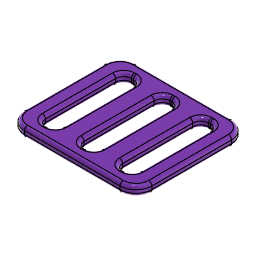
TriGlide v3 (Autodesk Fusion 360 design; units mm, degrees)
Autodesk Fusion 360 part; units mm, degrees
other "Base Mesh Feature1"
sketch "Sketch1" plane through (0, 0, 0) normal (0, 0, 1) x (1, 0, 0)
  line L0 (-12.5, 12.5) -> (-12.5, -12.5)
  line L1 (-7.5, -17.5) -> (22.5, -17.5)
  line L2 (27.5, -12.5) -> (27.5, 12.5)
  line L3 (22.5, 17.5) -> (-7.5, 17.5)
  arc A0 (-7.5, 17.5) -> (-12.5, 12.5) centre (-7.5, 12.5) ccw
  arc A1 (27.5, 12.5) -> (22.5, 17.5) centre (22.5, 12.5) ccw
  arc A2 (-12.5, -12.5) -> (-7.5, -17.5) centre (-7.5, -12.5) ccw
  arc A3 (22.5, -17.5) -> (27.5, -12.5) centre (22.5, -12.5) ccw
  dimension "d1" = 5
  dimension "outerFillet" = 5
  dimension "d3" = 5
  dimension "d4" = 5
  dimension "d17" = 40
  dimension "d18" = 12.5
  constraint vertical L0
  constraint perpendicular L0 L1
  constraint perpendicular L1 L2
  constraint perpendicular L2 L3
  constraint tangent L0 A0
  constraint tangent L3 A0
  constraint tangent L2 A1
  constraint tangent L3 A1
  constraint tangent L0 A2
  constraint tangent L1 A2
  constraint tangent L1 A3
  constraint tangent L2 A3
  measures "d1" radius of A0
  measures "outerFillet" radius of A1
  measures "d3" radius of A2
  measures "d4" radius of A3
  measures "d17" distance of L0 L2
  measures "d18" distance of origin L0
sketch "Sketch2" plane through (0, 0, 0) normal (0, 0, 1) x (1, 0, 0)
  line L0 (-4.9, 13.5) -> (-4.3, 13.5)
  line L1 (-4.9, -13.5) -> (-4.3, -13.5)
  line L2 (-7.4, 11) -> (-7.4, -11)
  line L3 (-1.8, -11) -> (-1.8, 11)
  arc A0 (-4.9, 13.5) -> (-7.4, 11) centre (-4.9, 11) ccw
  arc A1 (-1.8, 11) -> (-4.3, 13.5) centre (-4.3, 11) ccw
  arc A2 (-7.4, -11) -> (-4.9, -13.5) centre (-4.9, -11) ccw
  arc A3 (-4.3, -13.5) -> (-1.8, -11) centre (-4.3, -11) ccw
  dimension "d21" = 2.5
  dimension "d22" = 2.5
  dimension "d23" = 2.5
  dimension "d24" = 2.5
  dimension "d25" = 7.4
  dimension "d26" = 5.6
  constraint perpendicular L1 L2
  constraint perpendicular L0 L3
  constraint tangent L0 A0
  constraint tangent L2 A0
  constraint tangent L0 A1
  constraint tangent L3 A1
  constraint tangent L1 A2
  constraint tangent L2 A2
  constraint tangent L1 A3
  constraint tangent L3 A3
  measures "d21" radius of A0
  measures "d22" radius of A1
  measures "d23" radius of A2
  measures "d24" radius of A3
  measures "d25" distance of origin L2
  measures "d26" distance of L2 L3
extrude "Extrude1" add sketch "Sketch1" along normal blind 3 makes body 1
extrude "Extrude2" add sketch "Sketch2" along normal blind 3 separate body makes body 2
pattern_linear "R-Pattern1" count 3 spacing 12.1 along (1, 0, 0) of bodies 2 makes body 3 at (8.4333, -3.6667, 0) makes body 4 at (20.5333, -3.6667, 0)
combine "Combine1" operation cut target body 1 tool bodies 2 3 4
fillet "Fillet1" radius 1 16 edges at (27.5, 0, 0) (26.0355, 16.0355, 0) (7.5, 17.5, 0) (-11.0355, 16.0355, 0) (-12.5, 0, 0) (-11.0355, -16.0355, 0) (7.5, -17.5, 0) (26.0355, -16.0355, 0) (27.5, 0, 3) (26.0355, 16.0355, 3) (7.5, 17.5, 3) (-11.0355, 16.0355, 3) (-12.5, 0, 3) (-11.0355, -16.0355, 3) (7.5, -17.5, 3) (26.0355, -16.0355, 3) on bodies 1
fillet "Fillet2" radius 1 48 edges at (-4.6, -13.5, 3) (-6.6678, -12.7678, 3) (-7.4, 0, 3) (-6.6678, 12.7678, 3) (-4.6, 13.5, 3) (-2.5322, 12.7678, 3) (-1.8, 0, 3) (-2.5322, -12.7678, 3) (-6.6678, 12.7678, 0) (-7.4, 0, 0) (-6.6678, -12.7678, 0) (-4.6, -13.5, 0) (-2.5322, -12.7678, 0) (-1.8, 0, 0) (-2.5322, 12.7678, 0) (-4.6, 13.5, 0) (5.4322, -12.7678, 0) (7.5, -13.5, 0) (9.5678, -12.7678, 0) (10.3, 0, 0) (9.5678, 12.7678, 0) (7.5, 13.5, 0) (5.4322, 12.7678, 0) (4.7, 0, 0) (9.5678, 12.7678, 3) (10.3, 0, 3) (9.5678, -12.7678, 3) (7.5, -13.5, 3) (5.4322, -12.7678, 3) (4.7, 0, 3) (5.4322, 12.7678, 3) (7.5, 13.5, 3) (17.5322, 12.7678, 0) (16.8, 0, 0) (17.5322, -12.7678, 0) (19.6, -13.5, 0) (21.6678, -12.7678, 0) (22.4, 0, 0) (21.6678, 12.7678, 0) (19.6, 13.5, 0) (21.6678, -12.7678, 3) (19.6, -13.5, 3) (17.5322, -12.7678, 3) (16.8, 0, 3) (17.5322, 12.7678, 3) (19.6, 13.5, 3) (21.6678, 12.7678, 3) (22.4, 0, 3) on bodies 1
equation "d1 = outerFillet"
equation "d3 = outerFillet"
equation "innerFillet = 2.5 mm"
equation "d21 = innerFillet"
equation "d22 = innerFillet"
equation "d23 = innerFillet"
equation "d24 = innerFillet"
